Autodesk Inventor part; units mm, degrees
(part 3 of 3)
  spline S299 degree 2 poles (0.4706, 37.3013) (0.1043, 37.3013) (-0.3301, 37.6854) (-0.3301, 37.995) knots 0 0 0 1 2 2 2
  spline S300 degree 2 poles (-0.3301, 37.995) (-0.3301, 38.1344) (-0.2491, 38.3499) (-0.1632, 38.4294) knots 0 0 0 1 2 2 2
  spline S301 degree 2 poles (-0.1632, 38.4294) (-0.0773, 38.5104) (0.1707, 38.5963) (0.3506, 38.5963) knots 0 0 0 1 2 2 2
  line L257 (0.3506, 38.5963) -> (0.4884, 38.5963)
  line L258 (0.4884, 38.5963) -> (0.4884, 37.5574)
  spline S302 degree 2 poles (0.4884, 37.5574) (0.7493, 37.5574) (1.0265, 37.82) (1.0265, 38.0533) knots 0 0 0 1 2 2 2
  spline S303 degree 2 poles (1.0265, 38.0533) (1.0265, 38.136) (0.9892, 38.2964) (0.96, 38.3613) knots 0 0 0 1 2 2 2
  spline S304 degree 2 poles (0.96, 38.3613) (0.9276, 38.4294) (0.8709, 38.5234) (0.8449, 38.5541) knots 0 0 0 1 2 2 2
  line L259 (0.8449, 38.5541) -> (0.8449, 38.5687)
  line L260 (0.8449, 38.5687) -> (1.1205, 38.5687)
  spline S305 degree 2 poles (1.1205, 38.5687) (1.1383, 38.525) (1.1902, 38.3921) (1.2047, 38.3402) knots 0 0 0 1 2 2 2
  spline S306 degree 2 poles (1.2047, 38.3402) (1.2258, 38.2673) (1.2469, 38.1473) (1.2469, 38.0566) knots 0 0 0 1 2 2 2
  spline S307 degree 2 poles (0.2955, 38.3499) (0.1934, 38.3467) (0.0443, 38.3046) (-0.0059, 38.264) knots 0 0 0 1 2 2 2
  spline S308 degree 2 poles (-0.0059, 38.264) (-0.0627, 38.2203) (-0.1226, 38.0825) (-0.1226, 37.9804) knots 0 0 0 1 2 2 2
  spline S309 degree 2 poles (-0.1226, 37.9804) (-0.1226, 37.8799) (-0.0627, 37.7389) (-0.0043, 37.6806) knots 0 0 0 1 2 2 2
  spline S310 degree 2 poles (-0.0043, 37.6806) (0.0556, 37.6238) (0.1999, 37.5655) (0.2955, 37.5574) knots 0 0 0 1 2 2 2
  line L261 (0.2955, 37.5574) -> (0.2955, 38.3499)
  point P0 (0, 0)
  constraints: 4 other
extrude "Extrusion13" add sketch "Sketch14" along normal blind 0.2
equation "\"d1\" = d0"
equation "\"d2\" = d0"
equation "\"d3\" = d0"
equation "\"d16\" = d15"
equation "\"d17\" = d15"
equation "\"d18\" = d15"
equation "\"d37\" = -d28 + 0.5 * d36 - 0.5 * d35"
equation "\"d40\" = d42"
equation "\"d41\" = d43"
equation "\"d81\" = d80"
equation "\"d82\" = d80"
equation "\"d83\" = d80"
equation "\"d61\" = d60"
equation "\"d62\" = 0.5 * d60"
equation "\"d63\" = 0.5 * d60"
equation "\"d64\" = 0.5 * d60"
equation "\"d65\" = 0.5 * d60"
body "Solid1"
